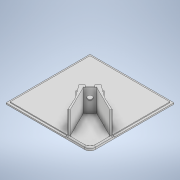
# Autodesk Inventor part: Box_Walls_2
Saved by Autodesk Inventor 2022 (Build 260153000, 153)
## iProperties
Created: 2023-02-27
Part Number: Box_Walls_2
Material: Generic
Document SubType Name: Modeling
Designer: zarek
Density: 1 g/cm^3
Appearance: Default
Author: zarek
Autodesk Inventor part; units mm, degrees
ref_plane "YZ Plane" through (0, 0, 0) normal (1, 0, 0) x (0, 1, 0)
ref_plane "XZ Plane" through (0, 0, 0) normal (0, 1, 0) x (-1, 0, 0)
sketch "Sketch1" plane through (0, 0, 0) normal (0, 1, 0) x (-1, 0, 0)
  line L0 (101.6, -101.6) -> (-101.6, -101.6)
  line L1 (-101.6, -101.6) -> (-101.6, 101.6)
  line L2 (-101.6, 101.6) -> (101.6, 101.6)
  line L3 (101.6, 101.6) -> (101.6, -101.6)
  line L4 (96.6, -96.6) -> (-96.6, -96.6)
  line L5 (-96.6, -96.6) -> (-96.6, 96.6)
  line L6 (-96.6, 96.6) -> (96.6, 96.6)
  line L7 (96.6, 96.6) -> (96.6, -96.6)
  line L8 (101.6, 101.6) -> (-40.4, 101.6)
  circle A0 centre (0, 0) radius 88.9
  circle A1 centre (0, 0) radius 109.337642
  line L9 (-40.4, 101.6) -> (-101.6, 40.4)
  line L10 (-45.4, 101.6) -> (-101.6, 45.4)
  line L11 (96.6, 96.6) -> (96.6, 101.6)
  line L12 (-45.4, 101.6) -> (-35.4, 101.6)
  line L13 (-35.4, 101.6) -> (-35.4, 96.6)
  line L14 (-35.4, 96.6) -> (-45.4, 96.6)
  line L15 (-45.4, 96.6) -> (-45.4, 101.6)
  line L16 (-45.4, 101.6) -> (-43.114, 101.6)
  line L17 (-43.114, 101.6) -> (-43.114, 96.6)
  line L18 (-43.114, 96.6) -> (-45.4, 96.6)
  line L19 (-45.4, 96.6) -> (-45.4, 101.6)
  line L20 (-96.6, 45.4) -> (-101.6, 45.4)
  line L21 (-101.6, 45.4) -> (-101.6, 43.114)
  line L22 (-101.6, 43.114) -> (-96.6, 43.114)
  line L23 (-96.6, 43.114) -> (-96.6, 45.4)
  point P0 (96.6, 51.216794)
  point P1 (101.6, 40.4)
  point P2 (101.6, -40.4)
  point P3 (96.6, -51.216794)
  point P4 (-96.6, 45.4)
  point P5 (-45.4, 96.6)
  dimension "d0" = 203.2
  dimension "d1" = 203.2
  dimension "d2" = 101.6
  dimension "d3" = 101.6
  dimension "d4" = 5
  dimension "d5" = 5
  dimension "d6" = 5
  dimension "d7" = 5
  dimension "d10" = 142
  dimension "d12" = 61.2
  dimension "d14" = 177.8
  dimension "d15" = 5
  dimension "d16" = 5
  dimension "d17" = 10
  dimension "d86" = 2.286
  dimension "d87" = 2.286
  constraints: 48 end point, 11 parallel, 10 point on line, 6 perpendicular, 5 horizontal, 2 centre point, 2 coincident, 2 point on circle
  measures "d0" distance between parallel lines of L2 L0
  measures "d1" distance between parallel lines of L1 L3
  measures "d2" distance from line of L0 point (0, 0)
  measures "d3" distance from line of L1 point (0, 0)
  measures "d4" distance between parallel lines of L4 L0
  measures "d5" distance between parallel lines of L1 L5
  measures "d6" distance between parallel lines of L2 L6
  measures "d7" distance between parallel lines of L3 L7
  measures "d10" distance of L2.end L8.end
  measures "d12" distance from line of L1 L8.end
  measures "d14" diameter of A0
  measures "d15" distance of L10.end L9.end
  measures "d16" distance of L10.start L8.end
  measures "d17" distance of L13.end L14.end
  measures "d86" distance of L17.end L18.end
  measures "d87" distance of L21.end L20.end
sketch "Sketch1 outline for Extrusion1" plane through (0, 0, 0) normal (0, 1, 0) x (-1, 0, 0)
  line L0 (-101.6, -101.6) -> (101.6, -101.6)
  line L1 (101.6, -101.6) -> (101.6, 101.6)
  line L2 (101.6, 101.6) -> (-101.6, 101.6)
  line L3 (-101.6, 101.6) -> (-101.6, -101.6)
extrude "Extrusion1" add sketch "Sketch1 outline for Extrusion1" along normal blind 5
sketch "Sketch3" plane through (0, 5, 0) normal (0, 1, 0) x (1, 0, 0)
  circle A0 centre (0, 0) radius 88.9
  line L0 (-101.6, 101.6) -> (-101.6, -101.6)
  line L1 (-101.6, -101.6) -> (101.6, -101.6)
  line L2 (-101.6, 101.6) -> (101.6, 101.6)
  line L3 (101.6, 101.6) -> (101.6, -101.6)
  line L4 (101.6, -101.6) -> (-101.6, -101.6)
  line L5 (-101.6, -101.6) -> (-101.6, 101.6)
  line L6 (-96.6, 96.6) -> (96.6, 96.6)
  line L7 (96.6, 96.6) -> (96.6, -96.6)
  line L8 (96.6, -96.6) -> (-96.6, -96.6)
  line L9 (-96.6, -96.6) -> (-96.6, 96.6)
  line L10 (-101.6, -101.6) -> (40.4, -101.6)
  circle A1 centre (0, 0) radius 109.337642
  line L11 (40.4, -101.6) -> (101.6, -40.4)
  line L12 (101.6, -101.6) -> (101.6, 101.6)
  line L13 (45.4038, -101.6) -> (101.6, -45.4038)
  line L14 (96.6, -45.4) -> (101.6, -45.4038)
  line L15 (45.4, -96.6) -> (45.4038, -101.6)
  line L16 (96.6, -45.4) -> (101.6, -45.4)
  line L17 (101.6, -45.4) -> (101.6, -43.114)
  line L18 (101.6, -43.114) -> (96.6, -43.114)
  line L19 (96.6, -43.114) -> (96.6, -45.4)
  line L20 (45.4038, -101.6) -> (43.1178, -101.6)
  line L21 (43.1178, -101.6) -> (43.1178, -96.6)
  line L22 (43.1178, -96.6) -> (45.4038, -96.6)
  line L23 (45.4038, -96.6) -> (45.4038, -101.6)
  point P0 (45.4038, -101.6)
  point P1 (50.4038, -96.6)
  point P2 (96.6, -50.4038)
  dimension "d28" = 177.8
  dimension "d29" = 5
  dimension "d30" = 5
  dimension "d31" = 5
  dimension "d32" = 5
  dimension "d33" = 142
  dimension "d76" = 5.0038
  dimension "d77" = 5.0038
  dimension "d88" = 2.286
  dimension "d89" = 2.286
  constraints: 42 end point, 10 point on line, 9 parallel, 4 horizontal, 4 perpendicular, 2 centre point, 2 coincident, 2 point on circle
  measures "d28" diameter of A0
  measures "d29" distance between parallel lines of L3 L7
  measures "d30" distance between parallel lines of L6 L2
  measures "d31" distance between parallel lines of L0 L9
  measures "d32" distance between parallel lines of L1 L8
  measures "d33" distance of L4.end L10.end
  measures "d76" distance of L13.end L11.end
  measures "d77" distance of L13.start L10.end
  measures "d88" distance of L17.end L16.end
  measures "d89" distance of L21.end L22.end
sketch "Sketch3 outline for Extrusion3" plane through (0, 5, 0) normal (0, 1, 0) x (1, 0, 0)
  line L0 (43.1178, -101.6) -> (43.1178, -96.6)
  line L1 (-101.6, -101.6) -> (43.1178, -101.6)
  line L2 (-101.6, 101.6) -> (-101.6, -101.6)
  line L3 (101.6, 101.6) -> (-101.6, 101.6)
  line L4 (101.6, -43.114) -> (101.6, 101.6)
  line L5 (96.6, -43.114) -> (101.6, -43.114)
  line L6 (96.6, 96.6) -> (96.6, -43.114)
  line L7 (-96.6, 96.6) -> (96.6, 96.6)
  line L8 (-96.6, -96.6) -> (-96.6, 96.6)
  line L9 (43.1178, -96.6) -> (-96.6, -96.6)
extrude "Extrusion3" cut sketch "Sketch3 outline for Extrusion3" against normal blind 2
sketch "Sketch4" plane through (0, 5, 0) normal (0, 1, 0) x (1, 0, 0)
  line L0 (101.6, 101.6) -> (-101.6, 101.6)
  line L1 (-101.6, 101.6) -> (-101.6, -101.6)
  line L2 (-101.6, -101.6) -> (101.6, -101.6)
  line L3 (101.6, -101.6) -> (101.6, 101.6)
  circle A0 centre (0, 0) radius 2.5
  line L4 (11.331386, 2.138998) -> (-2.138998, -11.331386)
  line L5 (0, 0) -> (-5.656854, 5.656854)
  line L6 (-5.656854, -14.849242) -> (-26.162951, 5.656855)
  line L7 (-5.656854, 26.162952) -> (14.849242, 5.656855)
  circle A1 centre (-5.656854, 5.656854) radius 14
  line L8 (-26.162951, 5.656855) -> (-5.656854, 26.162952)
  line L9 (14.849242, 5.656855) -> (-5.656854, -14.849242)
  line L10 (-40.305087, 5.656855) -> (-5.656854, 40.305087)
  line L11 (-5.656854, 40.305087) -> (28.991378, 5.656855)
  line L12 (28.991378, 5.656855) -> (-5.656854, -28.991377)
  line L13 (-5.656854, -28.991377) -> (-40.305087, 5.656855)
  line L14 (-22.645095, 9.174711) -> (-9.174711, 22.645095)
  line L15 (-9.174711, 22.645095) -> (-12.766813, 26.237197)
  line L16 (-12.766813, 26.237197) -> (-26.237197, 12.766813)
  line L17 (-26.237197, 12.766813) -> (-22.645095, 9.174711)
  point P0 (9.525, 22.5)
  point P1 (-9.525, -6.5)
  dimension "d37" = 203.2
  dimension "d38" = 203.2
  dimension "d39" = 8
  dimension "d40" = 28
  dimension "d41" = 29
  dimension "d42" = 29
  dimension "d43" = 14.5
  dimension "d44" = 10
  dimension "d45" = 10
  dimension "d46" = 10
  dimension "d47" = 10
  dimension "d48" = 5.08
  dimension "d49" = 9.525
  dimension "d50" = 9.525
  dimension "d55" = 101.6
  dimension "d56" = 101.6
  constraints: 36 end point, 8 parallel, 4 perpendicular, 2 centre point, 2 coincident, 2 point on line, 1 horizontal
  measures "d37" distance between parallel lines of L2 L0
  measures "d38" distance between parallel lines of L1 L3
  measures "d39" distance of L5.start L5.end
  measures "d40" diameter of A1
  measures "d41" distance between parallel lines of L9 L8
  measures "d42" distance between parallel lines of L7 L6
  measures "d43" distance from line of A1.centre L8
  measures "d44" distance between parallel lines of L11 L7
  measures "d45" distance between parallel lines of L8 L10
  measures "d46" distance between parallel lines of L13 L6
  measures "d47" distance between parallel lines of L12 L9
  measures "d48" distance between parallel lines of L14 L16
  measures "d49" distance from line of A1.centre L15
  measures "d50" distance from line of L5.end L17
  measures "d55" distance from line of point (0, 0) L1
  measures "d56" distance from line of L0 point (0, 0)
sketch "Sketch4 outline for Extrusion4" plane through (0, 5, 0) normal (0, 1, 0) x (1, 0, 0)
  line L0 (-40.305087, 5.656855) -> (-5.656854, -28.991377)
  line L1 (-5.656854, 40.305087) -> (-40.305087, 5.656855)
  line L2 (28.991378, 5.656855) -> (-5.656854, 40.305087)
  line L3 (-5.656854, -28.991377) -> (28.991378, 5.656855)
extrude "Extrusion4" cut sketch "Sketch4 outline for Extrusion4" against normal blind 1
sketch "Sketch6" plane through (0, 5, 0) normal (0, 1, 0) x (1, 0, 0)
  line L0 (45.4038, -101.6) -> (0, 0)
  line L1 (50.4038, -96.6) -> (45.4038, -101.6)
  line L2 (96.6, -43.114) -> (96.6, 96.6)
  line L3 (101.6, -101.6) -> (101.6, 101.6)
  circle A0 centre (0, 0) radius 34.925
  circle A1 centre (0, 0) radius 33.425
  line L4 (-101.6, 101.6) -> (-101.6, -101.6)
  line L5 (-101.6, -101.6) -> (40.4, -101.6)
  line L6 (-101.6, -101.6) -> (101.6, -101.6)
  line L7 (101.6, 101.6) -> (101.6, -43.114)
  line L8 (101.6, -45.4038) -> (0, 0)
  line L9 (-96.6, -96.6) -> (43.1178, -96.6)
  line L10 (96.6, -43.114) -> (96.6, 96.6)
  line L11 (43.1178, -101.6) -> (-101.6, -101.6)
  line L12 (101.6, -45.4038) -> (96.6, -50.4038)
  line L13 (45.4038, -101.6) -> (101.6, -45.4038)
  line L14 (43.1178, -101.6) -> (101.6, -101.6)
  line L15 (0, 0) -> (101.6, -50.4076)
  line L16 (50.4076, -101.6) -> (0, 0)
  line L17 (43.169361, -96.6) -> (47.926911, -96.6)
  line L18 (96.6, -43.169361) -> (96.6, -47.926911)
  line L19 (40.4, -101.6) -> (101.6, -40.4)
  point P0 (13.637413, -30.516415)
  point P1 (30.516415, -13.637413)
  point P2 (14.249414, -31.885888)
  point P3 (31.286053, -15.522194)
  point P4 (29.942343, -14.855528)
  point P5 (31.885888, -14.249414)
  point P6 (98.255522, -48.748278)
  point P7 (96.6, -47.926911)
  point P8 (47.926911, -96.6)
  point P9 (15.522194, -31.286053)
  point P10 (96.6, -45.4)
  point P11 (45.4, -96.6)
  point P12 (14.855528, -29.942343)
  point P13 (96.6, -45.4)
  point P14 (45.4, -96.6)
  point P15 (45.4, -96.6)
  point P16 (47.088956, -94.911044)
  point P17 (94.911044, -47.088956)
  point P18 (96.6, -45.4)
  point P19 (43.858319, -98.141681)
  point P20 (98.141681, -43.858319)
  point P21 (45.4, -96.6)
  point P22 (96.6, -45.4)
  dimension "d71" = 69.85
  dimension "d72" = 66.85
  dimension "d75" = 142
  dimension "d78" = 5.0038
  dimension "d82" = 5.0038
  constraints: 18 end point, 11 point on line, 2 centre point, 2 coincident, 1 collinear, 1 perpendicular
  measures "d71" diameter of A0
  measures "d72" diameter of A1
  measures "d75" distance of L4.end L5.end
  measures "d78" distance of L0.start L5.end
  measures "d82" distance of L8.start L19.end
sketch "Sketch6 outline for Extrusion6" plane through (0, 5, 0) normal (0, 1, 0) x (1, 0, 0)
  line L0 (45.4, -96.6) -> (47.088956, -94.911044)
  line L1 (43.169361, -96.6) -> (45.4, -96.6)
  line L2 (13.637413, -30.516415) -> (43.169361, -96.6)
  arc A0 (30.516415, -13.637413) -> (13.637413, -30.516415) centre (0, 0) cw
  line L3 (96.6, -43.169361) -> (30.516415, -13.637413)
  line L4 (96.6, -45.4) -> (96.6, -43.169361)
  line L5 (94.911044, -47.088956) -> (96.6, -45.4)
  line L6 (31.286053, -15.522194) -> (94.911044, -47.088956)
  arc A1 (15.522194, -31.286053) -> (31.286053, -15.522194) centre (0, 0) ccw
  line L7 (47.088956, -94.911044) -> (15.522194, -31.286053)
extrude "Extrusion6" add sketch "Sketch6 outline for Extrusion6" along normal blind 54.5
sketch "Sketch8" plane through (0, 5, 0) normal (0, 1, 0) x (1, 0, 0)
  line L0 (101.6, -101.6) -> (101.6, 101.6)
  line L1 (-96.6, -96.6) -> (43.1178, -96.6)
  line L2 (101.6, -101.6) -> (43.1178, -101.6)
  line L3 (43.1178, -101.6) -> (43.1178, -96.6)
  line L4 (43.1178, -96.6) -> (101.6, -96.6)
  line L5 (101.6, -96.6) -> (101.6, -101.6)
  line L6 (96.6, -43.114) -> (96.6, 96.6)
  line L7 (101.6, -101.6) -> (96.6, -101.6)
  line L8 (96.6, -101.6) -> (96.6, -43.114)
  line L9 (96.6, -43.114) -> (101.6, -43.114)
  line L10 (101.6, -43.114) -> (101.6, -101.6)
  line L11 (96.6, -45.4) -> (94.911044, -47.088956)
  line L12 (47.088956, -94.911044) -> (15.522194, -31.286053)
  line L13 (43.1178, -101.6) -> (101.6, -101.6)
  line L14 (43.1178, -101.6) -> (-101.6, -101.6)
  line L15 (-101.6, -101.6) -> (40.4, -101.6)
  line L16 (101.601962, -101.604818) -> (-101.598038, -101.604818)
  line L17 (-101.598038, -101.604818) -> (-101.598038, 101.595182)
  line L18 (-101.598038, 101.595182) -> (101.601962, 101.595182)
  line L19 (101.601962, 101.595182) -> (101.601962, -101.604818)
  line L20 (96.601962, -96.604818) -> (-96.598038, -96.604818)
  line L21 (-96.598038, -96.604818) -> (-96.598038, 96.595182)
  line L22 (-96.598038, 96.595182) -> (96.601962, 96.595182)
  line L23 (96.601962, 96.595182) -> (96.601962, -96.604818)
  line L24 (101.601962, 101.595182) -> (-40.398038, 101.595182)
  circle A0 centre (0.001962, -0.004818) radius 88.9
  circle A1 centre (0.001962, -0.004818) radius 109.337642
  line L25 (-40.398038, 101.595182) -> (-101.598038, 40.395182)
  line L26 (-45.398038, 101.595182) -> (-101.598038, 45.395182)
  line L27 (96.601962, 96.595182) -> (96.601962, 101.595182)
  line L28 (-45.398038, 101.595182) -> (-35.398038, 101.595182)
  line L29 (-35.398038, 101.595182) -> (-35.398038, 96.595182)
  line L30 (-35.398038, 96.595182) -> (-45.398038, 96.595182)
  line L31 (-45.398038, 96.595182) -> (-45.398038, 101.595182)
  line L32 (43.1178, -96.6) -> (43.1178, -101.6)
  line L33 (43.1178, -100.4824) -> (43.1178, -101.6)
  line L34 (51.218756, -96.604818) -> (52.336356, -96.604818)
  line L35 (100.4824, -43.114) -> (101.6, -43.114)
  line L36 (96.601962, -51.221612) -> (96.601962, -52.339212)
  line L37 (43.1178, -101.6) -> (46.927797, -101.604818)
  line L38 (101.6, -43.114) -> (101.601962, -46.923999)
  line L39 (101.601962, -46.923999) -> (96.601962, -52.491612)
  line L40 (96.601962, -51.221612) -> (96.601962, -54.317383)
  line L41 (46.927797, -101.604818) -> (52.488756, -96.604818)
  line L42 (51.218756, -96.604818) -> (52.488756, -96.604818)
  point P0 (0, 0)
  point P1 (-96.598038, -96.6)
  point P2 (43.1178, -96.604818)
  point P3 (101.6, -46.926184)
  point P4 (46.933155, -101.6)
  dimension "d93" = 142
  dimension "d94" = 203.2
  dimension "d95" = 203.2
  dimension "d96" = 101.6
  dimension "d97" = 101.6
  dimension "d98" = 5
  dimension "d99" = 5
  dimension "d100" = 5
  dimension "d101" = 5
  dimension "d102" = 142
  dimension "d103" = 61.2
  dimension "d104" = 177.8
  dimension "d105" = 5
  dimension "d106" = 5
  dimension "d107" = 10
  dimension "d116" = 3.81
  dimension "d117" = 3.81
  dimension "d118" = 1.27
  dimension "d119" = 1.27
  constraints: 70 end point, 17 point on line, 13 parallel, 6 perpendicular, 6 point on circle, 5 horizontal, 2 centre point, 2 coincident, 2 collinear, 1 vertical
  measures "d93" distance of L14.end L15.end
  measures "d94" distance between parallel lines of L18 L16
  measures "d95" distance between parallel lines of L17 L19
  measures "d96" distance from line of L16 point (0.002, -0.005)
  measures "d97" distance from line of L17 point (0.002, -0.005)
  measures "d98" distance between parallel lines of L20 L16
  measures "d99" distance between parallel lines of L17 L21
  measures "d100" distance between parallel lines of L18 L22
  measures "d101" distance between parallel lines of L19 L23
  measures "d102" distance of L24.start L24.end
  measures "d103" distance from line of L17 L24.end
  measures "d104" diameter of A0
  measures "d105" distance of L26.end L25.end
  measures "d106" distance of L31.end L24.end
  measures "d107" distance of L30.start L31.start
  measures "d116" distance of L2.end L37.end
  measures "d117" distance of L9.end L38.end
  measures "d118" distance of L39.end L36.start
  measures "d119" distance of L41.end L34.start
sketch "Sketch8 outline for Extrusion7" plane through (0, 5, 0) normal (0, 1, 0) x (1, 0, 0)
  line L0 (101.6, -46.926184) -> (96.601962, -52.491612)
  line L1 (101.6, -101.6) -> (101.6, -46.926184)
  line L2 (46.933155, -101.6) -> (101.6, -101.6)
  line L3 (52.488756, -96.604818) -> (46.933155, -101.6)
  line L4 (96.601962, -96.604818) -> (52.488756, -96.604818)
  line L5 (96.601962, -52.491612) -> (96.601962, -96.604818)
extrude "Extrusion7" add sketch "Sketch8 outline for Extrusion7" along normal blind 3
fillet "Fillet3" radius 12.7 2 edges at (101.6, 4, 101.6) (96.602, 6.5, 96.6048)
fillet "Fillet4" radius 3.175 6 edges at (97.8803, 8, 97.8803) (101.6, 8, 67.9131) (67.9166, 8, 101.6) (92.8822, 8, 92.8851) (96.602, 8, 68.1982) (68.1954, 8, 96.6048)
sketch "Sketch9" plane through (0, 4, 0) normal (0, 1, 0) x (1, 0, 0)
  point P0 (0, 0)
sketch "Sketch10" plane through (0, 5, 0) normal (0, 1, 0) x (1, 0, 0)
  point P0 (0, 0)
ref_plane "Work Plane1" through (24.695704, 5, 24.695704) normal (0.7071068, 0, 0.7071068) x (0.7071068, 0, -0.7071068)
sketch "Sketch15" plane through (0, 5, 0) normal (0, 1, 0) x (1, 0, 0)
  line L0 (13.637413, -30.516415) -> (43.169361, -96.6)
  line L1 (28.403387, -63.558207) -> (-0.656854, -23.991377)
  line L2 (28.991378, 5.656855) -> (-5.656854, -28.991377)
  line L3 (96.6, -43.169361) -> (30.516415, -13.637413)
  line L4 (-5.656854, 40.305087) -> (28.991378, 5.656855)
  line L5 (63.558207, -28.403387) -> (23.991378, 0.656855)
  line L6 (2.337401, -28.06819) -> (28.068191, -2.3374)
  arc A0 (13.637413, -30.516415) -> (30.516415, -13.637413) centre (0, 0) ccw
  line L7 (28.403387, -63.558207) -> (13.637413, -30.516415)
  line L8 (63.558207, -28.403387) -> (30.516415, -13.637413)
  arc A1 (13.637413, -30.516415) -> (30.516415, -13.637413) centre (0, 0) ccw
  dimension "d138" = 5
  dimension "d139" = 5
  dimension "d140" = 5
  constraints: 10 end point, 4 point on line, 3 point on circle, 2 midpoint, 1 centre point, 1 collinear, 1 concentric, 1 parallel
  measures "d138" horizontal distance of L2.end L1.end
  measures "d139" horizontal distance of L2.start L5.end
  measures "d140" distance between parallel lines of L6 L2
sketch "Sketch15 outline for Extrusion11" plane through (0, 5, 0) normal (0, 1, 0) x (1, 0, 0)
  arc A0 (13.637413, -30.516415) -> (30.516415, -13.637413) centre (0, 0) ccw
  line L0 (28.403387, -63.558207) -> (13.637413, -30.516415)
  line L1 (2.337401, -28.06819) -> (28.403387, -63.558207)
  line L2 (28.068191, -2.3374) -> (2.337401, -28.06819)
  line L3 (63.558207, -28.403387) -> (28.068191, -2.3374)
  line L4 (30.516415, -13.637413) -> (63.558207, -28.403387)
extrude "Extrusion11" add sketch "Sketch15 outline for Extrusion11" along normal up to surface (54.5 mm away)
sketch "Sketch16" plane through (0, 59.5, 0) normal (0, 1, 0) x (1, 0, 0)
  line L0 (2.337401, -28.06819) -> (28.068191, -2.3374)
  line L1 (9.408468, -20.997123) -> (12.944002, -24.532656)
  line L2 (12.944002, -24.532656) -> (24.532657, -12.944002)
  line L3 (24.532657, -12.944002) -> (20.997123, -9.408468)
  line L4 (12.944002, -24.532656) -> (24.532657, -12.944002)
  line L5 (24.532657, -12.944002) -> (28.559218, -16.970562)
  line L6 (28.559218, -16.970562) -> (16.970563, -28.559217)
  line L7 (16.970563, -28.559217) -> (12.944002, -24.532656)
  line L8 (12.944002, -24.532656) -> (5.331655, -32.145003)
  line L9 (28.403387, -63.558207) -> (2.337401, -28.06819)
  line L10 (24.532657, -12.944002) -> (32.145004, -5.331655)
  line L11 (28.068191, -2.3374) -> (63.558207, -28.403387)
  point P0 (0, 0)
  dimension "d144" = 10
  dimension "d145" = 10
  dimension "d146" = 5
  dimension "d152" = 0
  dimension "d153" = 0
  constraints: 18 end point, 6 perpendicular, 6 point on line
  measures "d144" distance of L0.start L1.start
  measures "d145" distance of L0.end L3.end
  measures "d146" distance between parallel lines of L0 L2
  measures "d152" distance between parallel lines of L7 L1
  measures "d153" distance between parallel lines of L5 L3
sketch "Sketch16 outline for Extrusion12" plane through (0, 59.5, 0) normal (0, 1, 0) x (1, 0, 0)
  line L0 (2.337401, -28.06819) -> (5.331655, -32.145003)
  line L1 (5.331655, -32.145003) -> (12.944002, -24.532656)
  line L2 (12.944002, -24.532656) -> (16.970563, -28.559217)
  line L3 (16.970563, -28.559217) -> (28.559218, -16.970562)
  line L4 (28.559218, -16.970562) -> (24.532657, -12.944002)
  line L5 (24.532657, -12.944002) -> (32.145004, -5.331655)
  line L6 (32.145004, -5.331655) -> (28.068191, -2.3374)
  line L7 (28.068191, -2.3374) -> (2.337401, -28.06819)
extrude "Extrusion12" cut sketch "Sketch16 outline for Extrusion12" against normal up to surface (54.5 mm away)
sketch "Sketch11" plane through (24.695704, 5, 24.695704) normal (0.7071068, 0, 0.7071068) x (0.7071068, 0, -0.7071068)
  line L0 (143.684098, -5) -> (0, -5)
  line L1 (0, -5) -> (0, 33.1)
  circle A0 centre (0, 33.1) radius 5.5
  dimension "d120" = 38.1
  dimension "d121" = 11
  constraints: 2 end point, 1 centre point, 1 coincident, 1 vertical
  measures "d120" distance of L0.end L1.end
  measures "d121" diameter of A0
sketch "Sketch11 outline for Extrusion8" plane through (24.695704, 5, 24.695704) normal (0.7071068, 0, 0.7071068) x (0.7071068, 0, -0.7071068)
  circle A0 centre (0, 33.1) radius 5.5
extrude "Extrusion8" cut sketch "Sketch11 outline for Extrusion8" against normal blind 127
sketch "Sketch17" plane through (5.331655, 5, 32.145003) normal (-0.7071068, 0, -0.7071068) x (-0.7071068, 0, 0.7071068)
  circle A0 centre (-18.987055, 33.097368) radius 3.428276
  line L0 (-13.587055, 38.396727) -> (-24.387055, 38.396727)
  line L1 (-24.387055, 38.396727) -> (-13.536096, 38.396727)
  line L2 (-13.536096, 38.396727) -> (-13.536096, 27.543561)
  line L3 (-13.536096, 27.543561) -> (-24.387055, 27.543561)
  line L4 (-24.387055, 27.543561) -> (-24.387055, 38.396727)
  line L5 (-8.087055, 23.634727) -> (-29.887055, 23.634727)
  line L6 (-28.13766, 47.496727) -> (-10.03645, 47.496727)
  line L7 (-6.487055, 44.415858) -> (-6.487055, 37.302596)
  line L8 (-31.487055, 37.571122) -> (-31.487055, 44.147332)
  circle A1 centre (-29.704997, 45.671817) radius 1.125053
  circle A2 centre (-8.441796, 45.671817) radius 1.129223
  circle A3 centre (-8.441796, 35.921088) radius 1.201492
  circle A4 centre (-29.704997, 35.921088) radius 1.201492
  circle A5 centre (-18.9599, 33.1) radius 5.5
  line L9 (-24.4599, 33.1) -> (-18.9599, 33.1)
  point P0 (-18.9599, -5)
  point P1 (-18.987055, 35.565727)
  dimension "d154" = 6.85655
  dimension "d155" = 10.85317
  dimension "d156" = 23.862
  dimension "d157" = 25
  dimension "d158" = 21.2632
  dimension "d159" = 9.75073
  dimension "d160" = 10.85096
  constraints: 20 end point, 5 centre point, 2 horizontal, 2 parallel, 1 horizontal alignment, 1 perpendicular, 1 other
  measures "d154" diameter of A0
  measures "d155" distance between parallel lines of L3 L0
  measures "d156" distance between parallel lines of L5 L6
  measures "d157" distance between parallel lines of L7 L8
  measures "d158" distance of A1.centre A2.centre
  measures "d159" distance of A1.centre A4.centre
  measures "d160" distance between parallel lines of L2 L4
hole "Hole1" at (26.33626, 50.671817, 11.140399) at (26.33626, 40.921088, 11.140399) at (11.300907, 50.671817, 26.175752) at (11.300907, 40.921088, 26.175752) direction (0.7071068, 0, 0.7071068) diameter 2.85 depth 5.08 tip angle 118 countersink diameter 3.048 countersink angle 82 thread size "M3.5x0.6" class "6H" standard "ANSI Metric M Profile"
equation "\"d1\" = d0"
equation "\"d2\" = 0.5 * d0"
equation "\"d3\" = 0.5 * d0"
equation "\"d95\" = d94"
equation "\"d96\" = 0.5 * d94"
equation "\"d97\" = 0.5 * d94"
body "Solid1"
